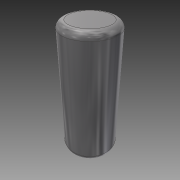
# Autodesk Inventor part: extruder_bearing_shaft
Saved by Autodesk Inventor 2014 (Build 180170000, 170)
## iProperties
Created: 2013-11-11
Part Number: extruder_bearing_shaft
Material: Stainless Steel, Austenitic
Document SubType Name: Modeling
Designer: buben
Density: 8.03 g/cm^3
Appearance: Semi-Polished
Mass: 7.99085 g
Surface Area: 5.80722 cm^2
Volume: 0.995125 cm^3
Author: buben
Autodesk Inventor part; units mm, degrees
ref_plane "YZ Plane" through (0, 0, 0) normal (1, 0, 0) x (0, 1, 0)
ref_plane "XZ Plane" through (0, 0, 0) normal (0, 1, 0) x (-1, 0, 0)
ref_plane "XY Plane" through (0, 0, 0) normal (0, 0, 1) x (1, 0, 0)
sketch "Sketch1" plane through (0, 0, 0) normal (0, 0, 1) x (1, 0, 0)
  circle A0 centre (0, 0) radius 4
  dimension "d0" = 8
  constraints: 1 centre point, 1 coincident
  measures "d0" diameter of A0
extrude "Extrusion1" add sketch "Sketch1" along normal blind 20
fillet "Fillet1" radius 1 2 edges at (-4, 0, 20) (-4, 0, 0)
body "Solid1"
